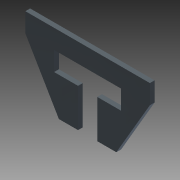
# Autodesk Inventor part: 5-1
Saved by Autodesk Inventor 2015 SP2 (Build 190223200, 223)
## iProperties
Created: 2015-09-23
Part Number: 5-1
Material: Iron, Cast
Document SubType Name: Modeling
Designer: Brandon
Density: 7.15 g/cm^3
Appearance: Iron Gray
Author: Brandon
Autodesk Inventor part; units mm, degrees
ref_plane "YZ Plane" through (0, 0, 0) normal (1, 0, 0) x (0, 1, 0)
ref_plane "XZ Plane" through (0, 0, 0) normal (0, 1, 0) x (-1, 0, 0)
ref_plane "XY Plane" through (0, 0, 0) normal (0, 0, 1) x (1, 0, 0)
sketch "Sketch1" plane through (0, 0, 0) normal (0, 0, 1) x (1, 0, 0)
  line L0 (0, 0) -> (165.1, 0)
  line L1 (165.1, 0) -> (165.1, -101.6)
  line L2 (165.1, -101.6) -> (0, -101.6)
  line L3 (0, -101.6) -> (0, 0)
  line L4 (0, -101.6) -> (44.45, -101.6)
  line L5 (0, -101.6) -> (0, -25.4)
  line L6 (0, -101.6) -> (69.85, -101.6)
  line L7 (69.85, -101.6) -> (69.85, -50.8)
  line L8 (69.85, -50.8) -> (38.1, -50.8)
  line L9 (38.1, -50.8) -> (38.1, -25.4)
  line L10 (38.1, -25.4) -> (127, -25.4)
  line L11 (127, -25.4) -> (127, -50.8)
  line L12 (127, -50.8) -> (95.25, -50.8)
  line L13 (95.25, -50.8) -> (95.25, -101.6)
  line L14 (165.1, -101.6) -> (120.65, -101.6)
  line L15 (165.1, -101.6) -> (165.1, -25.4)
  line L16 (165.1, -25.4) -> (120.65, -101.6)
  line L17 (0, -101.6) -> (0, -25.4)
  line L18 (0, -25.4) -> (44.45, -101.6)
  line L19 (44.45, -101.6) -> (0, -101.6)
  line L20 (0, -101.6) -> (0, -25.4)
  dimension "d0" = 165.1
  dimension "d4" = 44.45
  dimension "d5" = 69.85
  dimension "d10" = 25.4
  dimension "d11" = 25.4
  dimension "d12" = 101.6
  dimension "d13" = 38.1
  dimension "d14" = 25.4
  dimension "d15" = 44.45
  dimension "d17" = 88.9
  dimension "d18" = 165.1
  constraints: 42 end point, 8 perpendicular, 8 point on line, 3 equal length, 2 horizontal
  measures "d0" distance of L1.end L2.end
  measures "d4" distance of L2.end L4.end
  measures "d5" distance of L2.end L6.end
  measures "d10" distance of L12.end L7.end
  measures "d11" distance of L10.end L11.end
  measures "d12" distance of L2.end L0.start
  measures "d13" horizontal distance of L0.start L9.end
  measures "d14" distance from line of L0 L9.end
  measures "d15" distance of L1.end L14.end
  measures "d17" distance of L9.end L10.end
  measures "d18" distance of L0.start L0.end
extrude "Extrusion1" add sketch "Sketch1" along normal blind 6.35 contours L0 L1 L16 L2 L13 L12 L11 L10 L9 L8 L7 L18 L3
body "Solid1"
